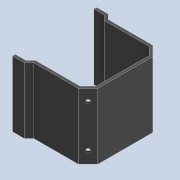
# Autodesk Inventor part: Z Axis Cover Bottom
Saved by Autodesk Inventor 2022 (Build 260153000, 153)
## iProperties
Created: 2021-10-26
Part Number: Z Axis Cover Bottom
Material: Generic
Document SubType Name: Modeling
Designer: Coy
Density: 1 g/cm^3
Appearance: Generic
Author: Coy
Autodesk Inventor part; units mm, degrees
ref_plane "YZ Plane" through (0, 0, 0) normal (1, 0, 0) x (0, 1, 0)
ref_plane "XZ Plane" through (0, 0, 0) normal (0, 1, 0) x (-1, 0, 0)
sketch "Sketch1" plane through (0, 0, 0) normal (0, 1, 0) x (-1, 0, 0)
  line L0 (0, 0) -> (0, 68.2)
  line L1 (0, 68.2) -> (10.6066, 78.8066)
  line L2 (10.6066, 78.8066) -> (68.3066, 78.8066)
  line L3 (68.3066, 78.8066) -> (74.5, 85)
  line L4 (74.5, 85) -> (88, 85)
  line L5 (0, 34.1) -> (80, 34.1) construction
  line L6 (0, 0) -> (10.6066, -10.6066)
  line L7 (10.6066, -10.6066) -> (68.3066, -10.6066)
  line L8 (68.3066, -10.6066) -> (74.5, -16.8)
  line L9 (74.5, -16.8) -> (88, -16.8)
  line L10 (88, 88.5) -> (73.0503, 88.5)
  line L11 (73.0503, 88.5) -> (66.8569, 82.3066)
  line L12 (66.8569, 82.3066) -> (9.1569, 82.3066)
  line L13 (9.1569, 82.3066) -> (-3.5, 69.6497)
  line L14 (-3.5, 69.6497) -> (-3.5, -1.4497)
  line L15 (-3.5, -1.4497) -> (9.1569, -14.1066)
  line L16 (9.1569, -14.1066) -> (66.8569, -14.1066)
  line L17 (66.8569, -14.1066) -> (73.0503, -20.3)
  line L18 (73.0503, -20.3) -> (88, -20.3)
  line L19 (88, 88.5) -> (88, 85)
  line L20 (88, -16.8) -> (88, -20.3)
  dimension "d0" = 68.2
  dimension "d1" = 15
  dimension "d2" = 135
  dimension "d5" = 135
  dimension "d6" = 88
  dimension "d7" = 3.5
  dimension "d18" = 13.5
  dimension "d19" = 50.9
  constraints: 42 end point, 4 parallel, 4 symmetric about line, 2 perpendicular, 2 vertical, 1 collinear, 1 horizontal, 1 midpoint, 8 other
  measures "d0" distance of L0.start L0.end
  measures "d1" distance of L0.end L1.end
  measures "d2" angle of L0 L1
  measures "d5" angle of L3 L2
  measures "d6" horizontal distance of L0.start L4.end
  measures "d7" distance between parallel lines of L3 L11
  measures "d18" distance of L3.end L4.end
  measures "d19" distance between parallel lines of L5 L4
extrude "Extrusion1" add sketch "Sketch1" along normal blind 85
sketch "Sketch2" plane through (3.5, 0, 69.6497) normal (0.7071068, 0, 0.7071068) x (0.7071068, 0, -0.7071068)
  line L0 (-17.8995, 0) -> (0, 0) projected
  line L1 (0, 0) -> (0, 85) projected
  line L2 (-17.8995, 85) -> (0, 85) projected
  line L3 (-17.8995, 0) -> (-17.8995, 85) projected
  line L4 (-1.4497, 85) -> (-16.4497, 85) construction
  line L5 (-8.9497, 85) -> (-8.9497, 0) construction
  line L6 (-17.8995, 0) -> (0, 0) construction
  circle A0 centre (-8.9497, 70) radius 2.6
  circle A1 centre (-8.9497, 15) radius 2.6
  point P0 (46.7749, 0)
  dimension "d10" = 5.2
  dimension "d11" = 5.2
  dimension "d12" = 15
  dimension "d13" = 15
  constraints: 2 centre point, 2 end point, 2 midpoint, 2 point on line
  measures "d10" diameter of A0
  measures "d11" diameter of A1
  measures "d12" distance from line of L2 A0.centre
  measures "d13" distance from line of L0 A1.centre
extrude "Extrusion2" cut sketch "Sketch2" against normal up to next contours A0 | A1
ref_plane "Work Plane1" through (-88, 0, 34.1) normal (0, 0, 1) x (1, 0, 0)
mirror "Mirror1" about plane through (-88, 0, 34.1) normal (0, 0, 1) of "Extrusion2"
sketch "Sketch4" plane through (-10.6066, 0, 78.8066) normal (0, 0, -1) x (-1, 0, 0)
  line L0 (27.7, 12) -> (42.7, 12)
  line L1 (42.7, 12) -> (42.7, 0)
  line L2 (42.7, 0) -> (27.7, 0)
  line L3 (27.7, 0) -> (27.7, 12)
  line L4 (0, 85) -> (57.7, 85) projected
  line L5 (57.7, 0) -> (57.7, 85) projected
  line L6 (0, 0) -> (57.7, 0) projected
  point P0 (-10.6066, 0)
  dimension "d20" = 15
  dimension "d21" = 12
  dimension "d22" = 15
  constraints: 8 end point, 2 parallel, 1 collinear, 1 horizontal, 1 perpendicular
  measures "d20" distance of L1.end L2.end
  measures "d21" distance of L0.end L1.end
  measures "d22" distance between parallel lines of L5 L1
extrude "Extrusion4" add sketch "Sketch4" along normal blind 6
sketch "Sketch5" plane through (-53.3066, 0, 78.8066) normal (-1, 0, 0) x (0, 0, 1)
  line L0 (0, 12) -> (0, 0) projected
  line L1 (0, 12) -> (-6, 12) projected
  line L2 (-6, 0) -> (-6, 12) projected
  line L3 (0, 0) -> (-6, 0) projected
  line L4 (-3.75, 7) -> (-2.25, 7)
  line L5 (-2.25, 7) -> (-2.25, 5)
  line L6 (-2.25, 5) -> (-3.75, 5)
  line L7 (-3.75, 5) -> (-3.75, 7)
  line L8 (-6, 0) -> (-6, 12) construction
  line L9 (-6, 6) -> (-3.75, 6) construction
  line L10 (0, 12) -> (-6, 12) construction
  line L11 (-3, 12) -> (-3, 7) construction
  point P0 (-78.8066, 0)
  dimension "d25" = 1.5
  dimension "d26" = 2
  constraints: 12 end point, 4 midpoint, 2 horizontal, 2 parallel, 2 perpendicular
  measures "d25" distance of L5.end L6.end
  measures "d26" distance of L4.end L5.end
extrude "Extrusion5" cut sketch "Sketch5" against normal up to next contours L4 L5 L6 L7
chamfer "Chamfer1" distance 3 distance2 6 1 edges at (-53.3066, 6, 72.8066) measured on face at (-43.3066, 8, 72.8066)
chamfer "Chamfer2" distance 3 distance2 6 1 edges at (-38.3066, 6, 72.8066) measured on face at (-42.3066, 8, 72.8066)
fillet "Fillet1" radius 6 2 edges at (-45.8066, 12, 72.8066) (-45.8066, 0, 72.8066)
equation "\"d11\" = d10"
equation "\"d13\" = d12"
body "Solid1"
